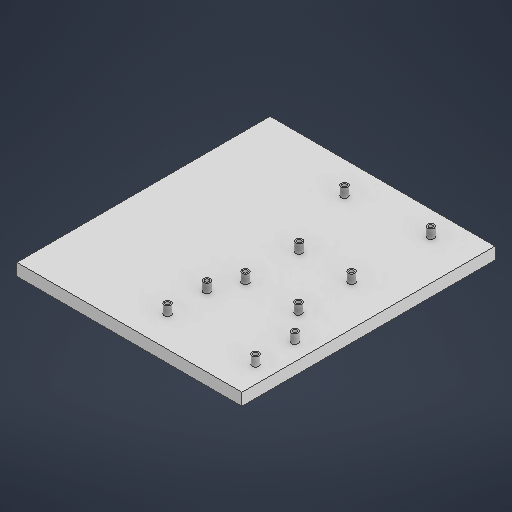
# Autodesk Inventor part: house
Saved by Autodesk Inventor 2026.2 (Build 302298000, 298)
## iProperties
Created: 2026-04-11
Part Number: house
Material: Generic
Document SubType Name: Modeling
Designer: Brian Wang
Density: 1 g/cm^3
Appearance: Default
Author: Brian Wang
Autodesk Inventor part; units mm, degrees
ref_plane "YZ Plane" through (0, 0, 0) normal (1, 0, 0) x (0, 1, 0)
ref_plane "XZ Plane" through (0, 0, 0) normal (0, 1, 0) x (-1, 0, 0)
ref_plane "XY Plane" through (0, 0, 0) normal (0, 0, 1) x (1, 0, 0)
sketch "Sketch1" plane through (0, 0, 0) normal (0, 1, 0) x (-1, 0, 0)
  line L0 (7.9805, 145.1359) -> (-134.4195, 145.1359)
  line L1 (-134.4195, 145.1359) -> (-134.4195, -21.8641)
  line L2 (-134.4195, -21.8641) -> (7.9805, -21.8641)
  line L3 (7.9805, -21.8641) -> (7.9805, 145.1359)
  line L4 (3.9805, 145.1359) -> (-50.0195, 145.1359)
  line L5 (-50.0195, 145.1359) -> (-50.0195, -21.8641)
  line L6 (-50.0195, -21.8641) -> (3.9805, -21.8641)
  line L7 (3.9805, -21.8641) -> (3.9805, 145.1359)
  line L8 (-126.2985, 137.7454) -> (-60.6985, 137.7454)
  line L9 (-60.6985, 137.7454) -> (-60.6985, 90.7454)
  line L10 (-60.6985, 90.7454) -> (-126.2985, 90.7454)
  line L11 (-126.2985, 90.7454) -> (-126.2985, 137.7454)
  line L12 (-67.0823, 41.9001) -> (-116.0823, 41.9001)
  line L13 (-116.0823, 41.9001) -> (-116.0823, 84.9001)
  line L14 (-116.0823, 84.9001) -> (-67.0823, 84.9001)
  line L15 (-67.0823, 84.9001) -> (-67.0823, 41.9001)
  line L16 (-127.0195, -15.0401) -> (-51.5195, -15.0401)
  line L17 (-51.5195, -15.0401) -> (-51.5195, 38.9599)
  line L18 (-51.5195, 38.9599) -> (-127.0195, 38.9599)
  line L19 (-127.0195, 38.9599) -> (-127.0195, -15.0401)
  circle A0 centre (-55.9195, -1.0401) radius 1.35
  circle A1 centre (-73.0247, 45.9001) radius 1.35
  circle A2 centre (-72.5195, 80.9001) radius 1.35
  circle A3 centre (-107.5195, 45.9001) radius 1.35
  circle A4 centre (-107.5195, 80.9001) radius 1.35
  circle A5 centre (-65.0195, 98.7881) radius 1.35
  circle A6 centre (-65.0195, 124.7881) radius 1.35
  circle A7 centre (-123.0195, 98.7881) radius 1.35
  circle A8 centre (-123.0195, 124.7881) radius 1.35
  circle A9 centre (-106.0195, 35.9599) radius 1.35
  point P0 (0, 0)
  point P1 (-63.2195, -21.8641)
  dimension "d0" = 142.4
  dimension "d1" = 167
  dimension "d2" = 54
  dimension "d3" = 4
  dimension "d21" = 47
  dimension "d22" = 49
  dimension "d23" = 43
  dimension "d25" = 54
  dimension "d27" = 77
  dimension "d29" = 2.7
  dimension "d31" = 14
  dimension "d32" = 71.1
  dimension "d33" = 2.7
  dimension "d34" = 2.7
  dimension "d35" = 2.7
  dimension "d36" = 2.7
  dimension "d52" = 2.7
  dimension "d53" = 2.7
  dimension "d54" = 26
  dimension "d55" = 2.7
  dimension "d56" = 2.7
  dimension "d57" = 26
  dimension "d59" = 58
  dimension "d60" = 15
  dimension "d77" = 2.7
  constraints: 40 end point, 10 centre point, 10 parallel, 6 horizontal, 5 perpendicular, 3 horizontal alignment, 2 point on line, 1 midpoint
  measures "d0" distance of L2.end L1.end
  measures "d1" distance of L2.end L0.start
  measures "d2" distance between parallel lines of L7 L5
  measures "d3" distance between parallel lines of L3 L7
  measures "d21" distance of L8.end L9.end
  measures "d22" distance of L13.end L14.end
  measures "d23" distance of L12.end L13.end
  measures "d25" distance of L17.end L16.end
  measures "d27" distance between parallel lines of L5 L19
  measures "d29" diameter of A0
  measures "d31" distance from line of L16 A0.centre
  measures "d32" distance from line of L19 A0.centre
  measures "d33" diameter of A1
  measures "d34" diameter of A2
  measures "d35" diameter of A3
  measures "d36" diameter of A4
  measures "d52" diameter of A5
  measures "d53" diameter of A6
  measures "d54" distance of A5.centre A6.centre
  measures "d55" diameter of A7
  measures "d56" diameter of A8
  measures "d57" distance of A7.centre A8.centre
  measures "d59" distance of A5.centre A7.centre
  measures "d60" distance from line of L5 A5.centre
  measures "d77" diameter of A9
extrude "Extrusion1" add sketch "Sketch1" along normal blind 8 contours L3 L2 L7 L0 | L7 L2 L5 L0 | L5 L2 L1 L0 | L8 L9 L10 L11 | L12 L13 L14 L15 | L19 L18 L17 L16 | A9
sketch "Sketch2" plane through (-7.9805, 0, -21.8641) normal (-1, 0, 0) x (0, 0, 1)
  circle A0 centre (13.5, 4) radius 1.35
  circle A1 centre (153.5, 4) radius 1.35
  line L0 (167, 0) -> (167, 8) projected
  circle A2 centre (3.5, 4) radius 1.35
  circle A3 centre (163.5, 4) radius 1.35
  point P0 (21.8641, 0)
  dimension "d63" = 2.7
  dimension "d64" = 2.7
  dimension "d65" = 140
  dimension "d67" = 2.7
  dimension "d68" = 2.7
  dimension "d69" = 10
  dimension "d70" = 10
  constraints: 4 centre point
  measures "d63" diameter of A0
  measures "d64" diameter of A1
  measures "d65" distance of A1.centre A0.centre
  measures "d67" diameter of A2
  measures "d68" diameter of A3
  measures "d69" distance of A3.centre A1.centre
  measures "d70" distance of A0.centre A2.centre
extrude "Extrusion2" cut sketch "Sketch2" against normal blind 8
sketch "Sketch3" plane through (0, 8, 0) normal (0, 1, 0) x (1, 0, 0)
  circle A0 centre (107.9195, 6.0401) radius 1.35
  circle A1 centre (55.9195, 1.0401) radius 1.35 projected
  point P0 (0, 0)
  dimension "d78" = 2.7
  dimension "d79" = 5
  dimension "d80" = 52
  constraints: 1 centre point
  measures "d78" diameter of A0
  measures "d79" vertical distance of A1.centre A0.centre
  measures "d80" horizontal distance of A1.centre A0.centre
extrude "Extrusion3" cut sketch "Sketch3" against normal through all contours A0
sketch "Sketch4" plane through (0, 8, 0) normal (0, 1, 0) x (1, 0, 0)
  circle A0 centre (107.9195, 6.0401) radius 1.35 projected
  circle A1 centre (107.9195, 6.0401) radius 2.25
  circle A2 centre (107.5195, -45.9001) radius 1.35 projected
  circle A3 centre (107.5195, -45.9001) radius 2.25
  circle A4 centre (55.9195, 1.0401) radius 1.35 projected
  circle A5 centre (55.9195, 1.0401) radius 2.25
  circle A6 centre (73.0247, -45.9001) radius 1.35 projected
  circle A7 centre (73.0247, -45.9001) radius 2.25
  circle A8 centre (72.5195, -80.9001) radius 1.35 projected
  circle A9 centre (72.5195, -80.9001) radius 2.25
  circle A10 centre (107.5195, -80.9001) radius 1.35 projected
  circle A11 centre (107.5195, -80.9001) radius 2.25
  circle A12 centre (123.0195, -98.7881) radius 1.35 projected
  circle A13 centre (123.0195, -98.7881) radius 2.25
  circle A14 centre (65.0195, -98.7881) radius 1.35 projected
  circle A15 centre (65.0195, -98.7881) radius 2.25
  circle A16 centre (65.0195, -124.7881) radius 1.35 projected
  circle A17 centre (65.0195, -124.7881) radius 2.25
  circle A18 centre (123.0195, -124.7881) radius 1.35 projected
  circle A19 centre (123.0195, -124.7881) radius 2.25
  circle A20 centre (107.9195, 6.0401) radius 1.35
  circle A21 centre (107.5195, -45.9001) radius 1.35
  circle A22 centre (55.9195, 1.0401) radius 1.35
  circle A23 centre (73.0247, -45.9001) radius 1.35
  circle A24 centre (107.5195, -80.9001) radius 1.35
  circle A25 centre (72.5195, -80.9001) radius 1.35
  circle A26 centre (65.0195, -98.7881) radius 1.35
  circle A27 centre (123.0195, -98.7881) radius 1.35
  circle A28 centre (123.0195, -124.7881) radius 1.35
  circle A29 centre (65.0195, -124.7881) radius 1.35
  point P0 (0, 0)
  dimension "d83" = 4.5
  dimension "d84" = 4.5
  dimension "d85" = 4.5
  dimension "d86" = 4.5
  dimension "d87" = 4.5
  dimension "d88" = 4.5
  dimension "d89" = 4.5
  dimension "d90" = 4.5
  dimension "d91" = 4.5
  dimension "d92" = 4.5
  dimension "d93" = 2.7
  dimension "d94" = 2.7
  dimension "d95" = 2.7
  dimension "d96" = 2.7
  dimension "d97" = 2.7
  dimension "d98" = 2.7
  dimension "d99" = 2.7
  dimension "d100" = 2.7
  dimension "d101" = 2.7
  constraints: 20 centre point, 20 coincident, 1 concentric
  measures "d83" diameter of A1
  measures "d84" diameter of A3
  measures "d85" diameter of A5
  measures "d86" diameter of A7
  measures "d87" diameter of A9
  measures "d88" diameter of A11
  measures "d89" diameter of A13
  measures "d90" diameter of A15
  measures "d91" diameter of A17
  measures "d92" diameter of A19
  measures "d93" diameter of A21
  measures "d94" diameter of A22
  measures "d95" diameter of A23
  measures "d96" diameter of A24
  measures "d97" diameter of A25
  measures "d98" diameter of A26
  measures "d99" diameter of A27
  measures "d100" diameter of A28
  measures "d101" diameter of A29
extrude "Extrusion4" add sketch "Sketch4" along normal blind 6
sketch "Sketch5" plane through (-7.9805, 0, -21.8641) normal (-1, 0, 0) x (0, 0, 1)
  line L0 (167, 8) -> (0, 8) projected
  line L1 (0, 8) -> (167, 8)
  line L2 (167, 8) -> (167, 0)
  line L3 (167, 0) -> (0, 0)
  line L4 (0, 0) -> (0, 8)
  circle A0 centre (13.5, 4) radius 1.35 projected
  circle A1 centre (13.5, 4) radius 1.35
  circle A2 centre (3.5, 4) radius 1.35 projected
  circle A3 centre (3.5, 4) radius 1.35
  circle A4 centre (153.5, 4) radius 1.35 projected
  circle A5 centre (153.5, 4) radius 1.35
  circle A6 centre (163.5, 4) radius 1.35 projected
  circle A7 centre (163.5, 4) radius 1.35
  point P0 (21.8641, 0)
  constraints: 8 end point, 4 centre point, 4 coincident, 2 parallel, 1 horizontal, 1 perpendicular
extrude "Extrusion5" add sketch "Sketch5" along normal blind 6
body "Solid1"
